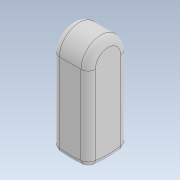
# Autodesk Inventor part: shank_link
Saved by Autodesk Inventor 2020 (Build 240168000, 168)
## iProperties
Created: 2020-12-22
Part Number: shank_link
Material: Generic
Document SubType Name: Modeling
Designer: DELL
Density: 1 g/cm^3
Appearance: Default
Author: DELL
Autodesk Inventor part; units mm, degrees
sketch "Sketch1" plane through (0, 0, 0) normal (1, 0, 0) x (0, 1, 0)
  line L0 (0, 0) -> (0, 25.2399) construction
  line L1 (0, 0) -> (0, -46.7601) construction
  line L2 (0, 0) -> (-120, 0) construction
  circle A0 centre (0, 0) radius 27.5
  line L3 (0, 27.5) -> (-120, 27.5)
  line L4 (0, -27.5) -> (-120, -27.5)
  line L5 (-120, 27.5) -> (-120, -27.5)
  line L6 (0, 0) -> (27.5, 0) construction
  circle A1 centre (0, 0) radius 120 construction
  arc A2 (-116.8065, 27.5) -> (-116.8065, -27.5) centre (0, 0) ccw
  line L7 (0, 0) -> (0, 27.5) construction
  line L8 (0, 0) -> (-120, 0)
  line L9 (-113.1371, 40) -> (-120, 40)
  line L10 (-120, 40) -> (-120, 0)
  arc A3 (-113.1371, 40) -> (-120, 0) centre (0, 0) ccw
  arc A4 (-20.1314, 27.5) -> (-20.1314, -27.5) centre (27.5, 0) ccw
  point P0 (-60, 0)
  point P1 (-120, 0)
  point P2 (-120, 27.5)
  point P3 (-116.8065, 27.5)
  dimension "d6" = 55
  dimension "d84" = 120
  dimension "d85" = 55
  dimension "d129" = 27.5
  dimension "d130" = 116.8065
  dimension "d131" = 3.1935
  dimension "d134" = 40
  dimension "d137" = 110
  constraints: 22 end point, 13 point on circle, 7 point on line, 5 centre point, 5 coincident, 2 collinear, 2 midpoint, 2 perpendicular, 2 tangent, 2 vertical, 1 horizontal, 1 symmetric about line, 1 other
  measures "d6" diameter of A0
  measures "d84" distance between parallel lines of L5 L1
  measures "d85" distance of L3.end L4.end
  measures "d129" distance from line of A1.end L2
  measures "d130" distance from line of L0 A1.end
  measures "d131" distance from line of L5 A1.end
  measures "d134" distance from line of L2.end L9
  measures "d137" diameter of A4
ref_plane "Work Plane1" through (14.5, 0, 0) normal (1, 0, 0) x (0, 1, 0)
ref_plane "Work Plane2" through (20, 0, 0) normal (1, 0, 0) x (0, 1, 0)
extrude "Extrusion4" add sketch "Sketch1" along normal mid plane 50 contours A0 | A0 A4 L3 | L4 A4 A0 | A4 L4 A2 L8 | L8 A2 L3 A4
revolve "Revolution1" cut sketch "Sketch1" angle 360 about axis through (0, 0, 0) along (0, -1, 0) contours L5 L3 A2 | L3 L10 L9 A3
sketch "Sketch6" plane through (0, 0, 0) normal (0, 1, 0) x (-1, 0, 0)
  circle A0 centre (0, 0) radius 10
  line L0 (-25, -27.5) -> (-25, 27.5) projected
  point P0 (-25, 27.5)
  point P1 (0, 0)
  dimension "d123" = 20
  constraints: 2 coincident, 1 centre point, 1 other
  measures "d123" diameter of A0
ref_plane "Work Plane5" through (0, -120, 0) normal (0, 1, 0) x (-1, 0, 0)
extrude "Extrusion11" cut sketch "Sketch6" along normal blind 60 from surface at -120
fillet "Fillet28" radius 10 5 edges at (25, 27.5, 0) (25, -57.0499, -27.5) (25, -57.0499, 27.5) (-25, -57.0499, 27.5) (-25, -57.0499, -27.5)
fillet "Fillet29" radius 8 7 edges at (25, -117.3669, 0) (0, -116.8065, -27.5) (-22.0815, -115.3654, -24.5606) (-25, -117.3669, 0) (-22.0815, -115.3654, 24.5606) (-7.5156, -116.5644, 27.5) (7.5156, -116.5644, 27.5)
body "Solid1"
